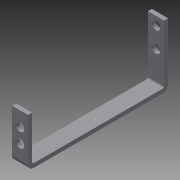
# Autodesk Inventor part: bottom pulley mount
Saved by Autodesk Inventor 2013 (Build 170138000, 138)
## iProperties
Created: 2013-02-07
Part Number: bottom pulley mount
Material: Generic
Document SubType Name: Sheet Metal
Designer: Arpan
Density: 1 g/cm^3
Sheet Metal Rule: Default
Mass: 7.12438 g
Surface Area: 60.3167 cm^2
Volume: 7.12438 cm^3
Flat Pattern Width: 1.27 cm
Flat Pattern Length: 18.7379 cm
Flat Pattern Area: 23.7971 cm^2
Sheet Metal Width: 0.500 in
Sheet Metal Length: 7.377 in
Sheet Metal Area: 3.689 in^2
Author: Arpan
Autodesk Inventor part; units mm, degrees
note: some values were not read from the file. Left out: dimensions or parameters whose unit could not be read.
ref_plane "YZ Plane" through (0, 0, 0) normal (1, 0, 0) x (0, 1, 0)
ref_plane "XZ Plane" through (0, 0, 0) normal (0, 1, 0) x (-1, 0, 0)
ref_plane "XY Plane" through (0, 0, 0) normal (0, 0, 1) x (1, 0, 0)
sketch "Sketch1" plane through (0, 0, 0) normal (0, 0, 1) x (1, 0, 0)
  line L0 (0, 0) -> (187.378778, 0)
  line L1 (187.378778, -12.7) -> (0, -12.7)
  line L2 (0, 0) -> (35.7378, 0)
  line L3 (35.7378, 0) -> (35.7378, -1.5875)
  line L4 (35.7378, -1.5875) -> (36.53155, -1.5875)
  line L5 (36.53155, -1.5875) -> (36.53155, 0)
  line L6 (35.7378, -1.5875) -> (34.94405, -1.5875)
  line L7 (34.94405, -1.5875) -> (34.94405, 0)
  line L8 (36.53155, -12.7) -> (34.94405, -12.7)
  line L9 (34.94405, -12.7) -> (34.94405, -11.1125)
  line L10 (34.94405, -11.1125) -> (36.53155, -11.1125)
  line L11 (36.53155, -11.1125) -> (36.53155, -12.7)
  line L12 (187.378778, 0) -> (151.640978, 0)
sketch "Sketch3" plane through (0, 0, 0) normal (0, 0, -1) x (-1, 0, 0)
  circle A0 centre (6.35164, 38.1) radius 3.3782
  circle A1 centre (6.35164, 22.225) radius 3.3782
sketch "Sketch6" plane through (-12.7, 33.655, 109.78515) normal (0, 0, 1) x (1, 0, 0)
  line L0 (0, 0) -> (12.7, 0)
  line L1 (0, -33.655) -> (0, 0)
  line L2 (6.35, 0) -> (6.35, -11.218333)
  line L3 (6.35, -11.218333) -> (6.35, -22.445133)
  circle A0 centre (6.35, -11.218333) radius 3.3782
  circle A1 centre (6.35, -22.445133) radius 3.3782
  dimension "d29" = 11.21833
  dimension "d31" = 11.2268
  dimension "d32" = 6.7564
  dimension "d33" = 6.7564
  constraints: 4 end point, 2 centre point, 2 coincident, 1 collinear, 1 midpoint, 1 parallel
  measures "d29" distance of L2.start L2.end
  measures "d31" distance of L2.end L3.end
  measures "d32" diameter of A0
  measures "d33" diameter of A1
sketch "Sketch1 outline for Plate1" plane through (0, 0, 0) normal (0, 0, 1) x (1, 0, 0)
  line L0 (0, 0) -> (-12.7, 0)
  line L1 (-12.7, 0) -> (-12.7, 44.45)
  line L2 (-12.7, 44.45) -> (0, 44.45)
  line L3 (0, 44.45) -> (0, 0)
extrude "Plate1" add sketch "Sketch1 outline for Plate1" along normal blind 3.175
sketch "Sketch2" plane through (0, -12.7, 0) normal (0, 0, 1) x (1, 0, 0)
  line L0 (35.7378, 11.1125) -> (35.7378, 12.7)
  line L1 (0, 12.7) -> (35.7378, 12.7)
  line L2 (36.53155, 12.7) -> (187.378778, 12.7)
  line L3 (35.7378, 11.1125) -> (34.94405, 11.1125)
  line L4 (34.94405, 11.1125) -> (34.94405, 12.7)
  constraints: 6 end point, 1 horizontal, 1 perpendicular, 1 vertical
edge flange "Flange1" height 105.34015 angle 90 thickness 3.175 bend radius 1.27 thickness toward (0, -1, 0) relief straight relief width 3.175 relief depth 1.5875 edges at (-6.35, 0, 3.175) wall of the first edge with corners at (-12.7, -1.27, 4.445) (0, -1.27, 4.445) (0, -1.27, 105.34015) (-12.7, -1.27, 105.34015)
bend "Bend1"
corner "Corner1"
sketch "Sketch4" plane through (0, -12.7, 0) normal (0, 0, 1) x (1, 0, 0)
  line L0 (187.378778, 0) -> (36.53155, 0)
  line L1 (36.53155, 12.7) -> (187.378778, 12.7)
  line L2 (187.378778, 12.7) -> (140.845978, 12.7)
  line L3 (140.845978, 12.7) -> (140.845978, 11.1125)
  line L4 (140.845978, 11.1125) -> (141.639728, 11.1125)
  line L5 (141.639728, 11.1125) -> (141.639728, 12.7)
  line L6 (140.845978, 11.1125) -> (140.052228, 11.1125)
  line L7 (140.052228, 11.1125) -> (140.052228, 12.7)
  line L8 (140.845978, 0) -> (141.639728, 0)
  line L9 (141.639728, 0) -> (141.639728, 1.5875)
  line L10 (141.639728, 1.5875) -> (140.052228, 1.5875)
  line L11 (140.052228, 1.5875) -> (140.052228, 0)
  dimension "d15" = 1.5875
  constraints: 20 end point, 6 perpendicular, 6 point on line, 2 parallel
  measures "d15" distance of L8.end L9.end
extrude "Cut1" cut sketch "Sketch3" against normal blind 3.175
sketch "Sketch5" plane through (0, -12.7, 0) normal (0, 0, 1) x (1, 0, 0)
  line L0 (140.845978, 12.7) -> (140.845978, 11.1125)
  line L1 (140.845978, 12.7) -> (187.378778, 12.7)
  line L2 (140.845978, 11.1125) -> (141.639728, 11.1125)
  line L3 (141.639728, 11.1125) -> (141.639728, 12.7)
  constraints: 6 end point, 1 horizontal, 1 perpendicular, 1 vertical
edge flange "Flange2" height 38.1 angle 90 thickness 3.175 bend radius 1.27 thickness toward (0, 0, 1) relief straight relief width 3.175 relief depth 1.5875 edges at (-6.35, -1.27, 105.34015) wall of the first edge with corners at (-12.7, 0, 106.61015) (0, 0, 106.61015) (0, 33.655, 106.61015) (-12.7, 33.655, 106.61015)
bend "Bend2"
corner "Corner2"
extrude "Cut3" cut sketch "Sketch6" against normal blind 3.175
equation "\"d3\" = BendReliefWidth"
equation "\"d4\" = BendReliefDepth"
equation "\"d5\" = MinimumRemnant"
equation "\"d6\" = BendRadius"
equation "\"d10\" = CornerReliefSize"
equation "\"d11\" = GapSize"
equation "\"d12\" = JacobiRadiusSize"
equation "\"d19\" = BendReliefWidth"
equation "\"d20\" = BendReliefDepth"
equation "\"d21\" = MinimumRemnant"
equation "\"d22\" = BendRadius"
equation "\"d26\" = CornerReliefSize"
equation "\"d27\" = GapSize"
equation "\"d28\" = JacobiRadiusSize"
equation "\"BendRadius\" = Thickness"
equation "\"BendReliefWidth\" = Thickness"
equation "\"BendReliefDepth\" = 0.5 * Thickness"
equation "\"CornerReliefSize\" = 4 * Thickness"
equation "\"MinimumRemnant\" = 2 * Thickness"
equation "\"TransitionRadius\" = BendRadius"
equation "\"JacobiRadiusSize\" = Thickness"
equation "\"GapSize\" = Thickness"
equation "\"d2\" = BendRadius"
equation "\"d6\" = Thickness"
equation "\"d16\" = Thickness"
equation "\"Thickness\" = 3.175"
body "Solid1"
